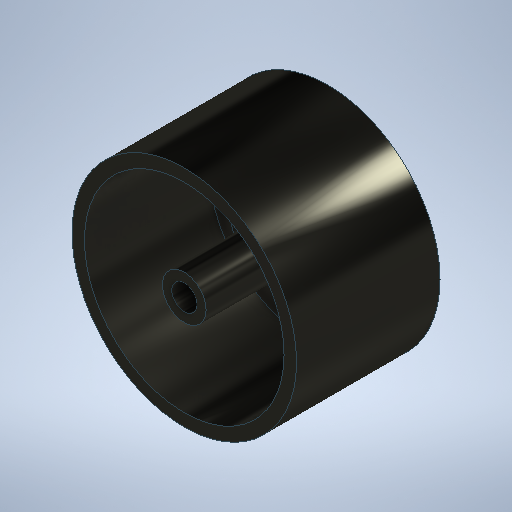
# Autodesk Inventor part: Electromagnet cover
Saved by Autodesk Inventor 2025 (Build 290162000, 162)
## iProperties
Created: 2026-07-22
Part Number: Electromagnet cover
Material: Generic
Document SubType Name: Sheet Metal
Designer: matot
Density: 1 g/cm^3
Sheet Metal Rule: Default_mm
Appearance: Expanded Metal 01
Author: matot
Autodesk Inventor part; units mm, degrees
ref_plane "YZ Plane" through (0, 0, 0) normal (1, 0, 0) x (0, 1, 0)
ref_plane "XZ Plane" through (0, 0, 0) normal (0, 1, 0) x (-1, 0, 0)
ref_plane "XY Plane" through (0, 0, 0) normal (0, 0, 1) x (1, 0, 0)
sketch "Sketch1" plane through (0, 0, 0) normal (0, 0, 1) x (1, 0, 0)
  circle A0 centre (0, 0) radius 90
  circle A1 centre (0, 0) radius 10
  dimension "d1" = 20
  dimension "d2" = 180
  constraints: 2 centre point, 2 coincident
  measures "d1" diameter of A1
  measures "d2" diameter of A0
extrude "Extrusion1" add sketch "Sketch1" along normal blind 15
sketch "Sketch2" plane through (0, 0, 15) normal (0, 0, 1) x (1, 0, 0)
  circle A0 centre (0, 55) radius 25
  circle A1 centre (-47.6314, 27.5) radius 25
  circle A2 centre (-47.6314, -27.5) radius 25
  circle A3 centre (0, -55) radius 25
  circle A4 centre (47.6314, -27.5) radius 25
  circle A5 centre (47.6314, 27.5) radius 25
  circle A6 centre (0, 55) radius 15
  circle A7 centre (-47.6314, 27.5) radius 15
  circle A8 centre (-47.6314, -27.5) radius 15
  circle A9 centre (0, -55) radius 15
  circle A10 centre (47.6314, -27.5) radius 15
  circle A11 centre (47.6314, 27.5) radius 15
  point P0 (0, 0)
  point P1 (0, 0)
  point P2 (0, 0)
  point P3 (0, 0)
  point P4 (0, 0)
  point P5 (0, 0)
  dimension "d5" = 50
  dimension "d6" = 55
  dimension "d9" = 360
  dimension "d11" = 30
  dimension "d14" = 360
  constraints: 12 centre point, 3 coincident, 30 other
  measures "d5" diameter of A0
  measures "d6" distance of point (0, 0) A0.centre
  measures "d11" diameter of A6
extrude "Extrusion2" cut sketch "Sketch2" against normal blind 15 contours A6 | A7 | A8 | A9 | A10 | A11
sketch "Sketch3" plane through (0, 0, 15) normal (0, 0, 1) x (1, 0, 0)
  circle A0 centre (0, 0) radius 90
  circle A1 centre (0, 0) radius 80
  dimension "d18" = 160
  dimension "d19" = 180
  constraints: 2 centre point, 2 coincident
  measures "d18" diameter of A1
  measures "d19" diameter of A0
extrude "Extrusion3" add sketch "Sketch3" along normal blind 100
sketch "Sketch4" plane through (0, 0, 15) normal (0, 0, 1) x (1, 0, 0)
  circle A0 centre (0, -54.6919) radius 25
  circle A1 centre (47.3646, -27.3459) radius 25
  circle A2 centre (47.3646, 27.3459) radius 25
  circle A3 centre (0, 54.6919) radius 25
  circle A4 centre (-47.3646, 27.3459) radius 25
  circle A5 centre (-47.3646, -27.3459) radius 25
  circle A6 centre (0, 0) radius 17.5
  circle A7 centre (0, 0) radius 10
  dimension "d22" = 50
  dimension "d25" = 360
  dimension "d27" = 35
  constraints: 8 centre point, 2 coincident, 13 other
  measures "d22" diameter of A0
  measures "d27" diameter of A6
extrude "Extrusion4" add sketch "Sketch4" along normal blind 100 contours A6 | A7
sketch "Sketch5" plane through (0, 0, 115) normal (0, 0, 1) x (1, 0, 0)
  circle A0 centre (0, 0) radius 10
  dimension "d30" = 20
  constraints: 1 centre point, 1 coincident
  measures "d30" diameter of A0
extrude "Extrusion5" cut sketch "Sketch5" against normal through all
equation "\"BendRadius\" = Thickness"
equation "\"BendReliefWidth\" = Thickness"
equation "\"BendReliefDepth\" = 0.5 * Thickness"
equation "\"CornerReliefSize\" = 4 * Thickness"
equation "\"MinimumRemnant\" = 2 * Thickness"
equation "\"TransitionRadius\" = BendRadius"
equation "\"JacobiRadiusSize\" = BendRadius"
equation "\"GapSize\" = Thickness"
equation "\"Thickness\" = 0.5"
body "Solid1"
